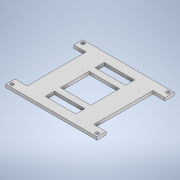
# Autodesk Inventor part: reg_board_plate
Saved by Autodesk Inventor 2020 (Build 240168000, 168)
## iProperties
Created: 2022-10-27
Part Number: reg_board_plate
Material: 일반
Document SubType Name: Modeling
Designer: SeungJin
Density: 1 g/cm^3
Appearance: 기본값
Author: SeungJin
Autodesk Inventor part; units mm, degrees
ref_plane "YZ Plane" through (0, 0, 0) normal (1, 0, 0) x (0, 1, 0)
ref_plane "XZ Plane" through (0, 0, 0) normal (0, 1, 0) x (-1, 0, 0)
ref_plane "XY Plane" through (0, 0, 0) normal (0, 0, 1) x (1, 0, 0)
sketch "스케치1" plane through (0, 0, 0) normal (0, 1, 0) x (-1, 0, 0)
  line L0 (70, 58.5) -> (-70, 58.5)
  line L1 (-70, 58.5) -> (-70, -58.5)
  line L2 (-70, -58.5) -> (70, -58.5)
  line L3 (70, -58.5) -> (70, 58.5)
  line L4 (70, 58.5) -> (-70, -58.5) construction
  line L5 (-70, 58.5) -> (70, -58.5) construction
  line L6 (75, -63.5) -> (-75, -63.5)
  line L7 (-75, -63.5) -> (-75, 63.5)
  line L8 (-75, 63.5) -> (75, 63.5)
  line L9 (75, 63.5) -> (75, -63.5)
  line L10 (75, -63.5) -> (-75, 63.5) construction
  line L11 (-75, -63.5) -> (75, 63.5) construction
  point P0 (0, 0)
  dimension "d0" = 140
  dimension "d1" = 117
  dimension "d2" = 150
  dimension "d3" = 127
  constraints: 24 end point, 4 midpoint, 4 parallel, 2 horizontal, 2 perpendicular
  measures "d0" distance of L2.end L1.end
  measures "d1" distance of L1.end L0.end
  measures "d2" distance of L7.end L8.end
  measures "d3" distance of L6.end L7.end
extrude "돌출1" add sketch "스케치1" along normal blind 5 contours L3 L2 L1 L0 | L6 L7 L8 L9
sketch "스케치2" plane through (0, 0, 0) normal (0, -1, 0) x (1, 0, 0)
  line L0 (-70, 58.5) -> (70, 58.5)
  line L1 (70, 58.5) -> (70, -58.5)
  line L2 (70, -58.5) -> (-70, -58.5)
  line L3 (-70, -58.5) -> (-70, 58.5)
  line L4 (-70, 58.5) -> (70, -58.5) construction
  line L5 (70, 58.5) -> (-70, -58.5) construction
  point P0 (0, 0)
  dimension "d6" = 140
  dimension "d7" = 117
  constraints: 12 end point, 2 midpoint, 2 parallel, 1 horizontal, 1 perpendicular
  measures "d6" distance of L1.end L2.end
  measures "d7" distance of L0.end L1.end
hole "구멍1" at (-70, 0, 58.5) at (70, 0, 58.5) at (-70, 0, -58.5) at (70, 0, -58.5) direction (0, 1, 0) diameter 5.5 end through all clearance for "Socket Head Cap Screw ISO 4762" size "M5" standard "ISO"
sketch "스케치3" plane through (0, 0, 0) normal (0, -1, 0) x (1, 0, 0)
  line L0 (-75, -63.5) -> (-75, 63.5) projected
  line L1 (75, 63.5) -> (75, -63.5) projected
  line L2 (75, -63.5) -> (-75, -63.5) projected
  line L3 (-75, 63.5) -> (75, 63.5) projected
  line L4 (-55, 48.5) -> (-55, -48.5)
  line L5 (75, -63.5) -> (-75, -63.5) projected
  line L6 (55, 48.5) -> (55, -48.5)
  line L7 (-25, 33.5) -> (25, 33.5)
  line L8 (-25, 23.5) -> (25, 23.5)
  line L9 (-25, -23.5) -> (25, -23.5)
  line L10 (-25, -33.5) -> (25, -33.5)
  line L11 (55, 48.5) -> (75, 48.5)
  line L12 (-75, 48.5) -> (-55, 48.5)
  line L13 (-25, 48.5) -> (25, 48.5)
  line L14 (-75, -48.5) -> (-55, -48.5)
  line L15 (-25, -48.5) -> (25, -48.5)
  line L16 (55, -48.5) -> (75, -48.5)
  line L17 (25, -33.5) -> (25, -48.5)
  line L18 (-25, -33.5) -> (-25, -48.5)
  line L19 (-25, 48.5) -> (-25, 33.5)
  line L20 (-25, 23.5) -> (-25, -23.5)
  line L21 (25, 48.5) -> (25, 33.5)
  line L22 (25, 23.5) -> (25, -23.5)
  point P0 (0, 0)
  dimension "d19" = 20
  dimension "d21" = 20
  dimension "d24" = 10
  dimension "d26" = 10
  dimension "d28" = 15
  dimension "d29" = 15
  dimension "d30" = 15
  dimension "d31" = 15
  dimension "d32" = 15
  dimension "d33" = 15
  dimension "d34" = 15
  dimension "d35" = 15
  dimension "d36" = 30
  dimension "d37" = 30
  dimension "d38" = 30
  dimension "d39" = 30
  dimension "d40" = 30
  dimension "d41" = 30
  constraints: 36 end point, 11 perpendicular, 3 horizontal, 2 point on line, 1 parallel
  measures "d19" distance between parallel lines of L0 L4
  measures "d21" distance between parallel lines of L1 L6
  measures "d24" distance between parallel lines of L7 L8
  measures "d26" distance between parallel lines of L9 L10
  measures "d28" distance between parallel lines of L2 L15
  measures "d29" distance between parallel lines of L7 L13
  measures "d30" distance between parallel lines of L15 L10
  measures "d31" distance between parallel lines of L3 L13
  measures "d32" distance between parallel lines of L3 L11
  measures "d33" distance between parallel lines of L3 L12
  measures "d34" distance between parallel lines of L5 L14
  measures "d35" distance between parallel lines of L2 L16
  measures "d36" distance between parallel lines of L6 L21
  measures "d37" distance between parallel lines of L22 L6
  measures "d38" distance between parallel lines of L17 L6
  measures "d39" distance between parallel lines of L4 L18
  measures "d40" distance between parallel lines of L4 L20
  measures "d41" distance between parallel lines of L4 L19
extrude "돌출2" cut sketch "스케치3" against normal blind 5 contours L0 L12 L4 L14 | L16 L6 L11 L1 | L19 L13 L21 L7 | L8 L22 L9 L20 | L10 L17 L15 L18
